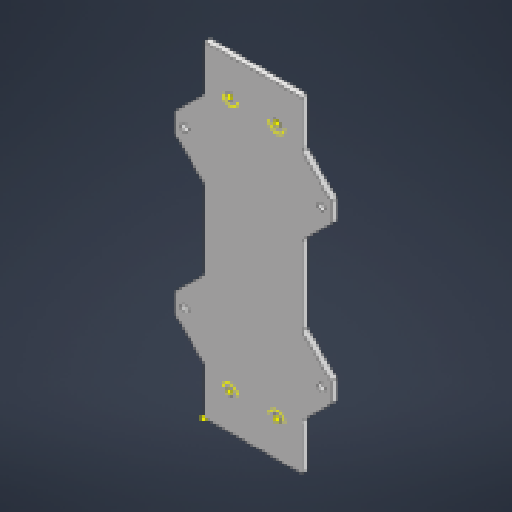
# Autodesk Inventor part: Center_lysekrone
Saved by Autodesk Inventor 2023.4 (Build 274418000, 418)
## iProperties
Created: 2025-10-22
Part Number: Center_lysekrone
Material: Generic
Document SubType Name: Modeling
Designer: Malthe Sennels
Density: 1 g/cm^3
Appearance: Default
Author: Malthe Sennels
Autodesk Inventor part; units mm, degrees
ref_plane "YZ Plane" through (0, 0, 0) normal (1, 0, 0) x (0, 1, 0)
ref_plane "XZ Plane" through (0, 0, 0) normal (0, 1, 0) x (-1, 0, 0)
ref_plane "XY Plane" through (0, 0, 0) normal (0, 0, 1) x (1, 0, 0)
sketch "Sketch1" plane through (0, 0, 0) normal (0, 0, 1) x (1, 0, 0)
  circle A0 centre (37, 149.0522) radius 1.75 projected
  circle A1 centre (13, 149.0522) radius 1.75 projected
  line L0 (50, 167.0522) -> (0, 167.0522) projected
  line L1 (0, 167.0522) -> (0, 157.0522) projected
  line L2 (7.8364, 157.0522) -> (0, 157.0522) construction
  line L3 (9.0389, 148.4955) -> (7.8364, 157.0522) construction
  arc A2 (9.0389, 148.4955) -> (16.9611, 148.4955) centre (13, 149.0522) ccw construction
  line L4 (18.1636, 157.0522) -> (16.9611, 148.4955) construction
  line L5 (31.8364, 157.0522) -> (18.1636, 157.0522) construction
  line L6 (33.0389, 148.4955) -> (31.8364, 157.0522) construction
  arc A3 (33.0389, 148.4955) -> (40.9611, 148.4955) centre (37, 149.0522) ccw construction
  line L7 (42.1636, 157.0522) -> (40.9611, 148.4955) construction
  line L8 (50, 157.0522) -> (42.1636, 157.0522) construction
  line L9 (50, 167.0522) -> (50, 157.0522) projected
  circle A4 centre (13, 18) radius 1.75 projected
  circle A5 centre (37, 18) radius 1.75 projected
  line L10 (0, 0) -> (50, 0) projected
  line L11 (50, 0) -> (50, 10) projected
  line L12 (42.1636, 10) -> (50, 10) construction
  line L13 (40.9611, 18.5567) -> (42.1636, 10) construction
  arc A6 (40.9611, 18.5567) -> (33.0389, 18.5567) centre (37, 18) ccw construction
  line L14 (31.8364, 10) -> (33.0389, 18.5567) construction
  line L15 (18.1636, 10) -> (31.8364, 10) construction
  line L16 (16.9611, 18.5567) -> (18.1636, 10) construction
  arc A7 (16.9611, 18.5567) -> (9.0389, 18.5567) centre (13, 18) ccw construction
  line L17 (7.8364, 10) -> (9.0389, 18.5567) construction
  line L18 (0, 10) -> (7.8364, 10) construction
  line L19 (0, 0) -> (0, 10) projected
  line L20 (0, 167.0522) -> (50, 167.0522)
  line L21 (50, 167.0522) -> (50, 0)
  line L22 (50, 0) -> (0, 0)
  line L23 (0, 0) -> (0, 167.0522)
  constraints: 8 end point, 2 parallel, 1 horizontal, 1 perpendicular
extrude "Extrusion1" add sketch "Sketch1" along normal blind 3
sketch "Sketch2" plane through (0, 0, 3) normal (0, 0, 1) x (1, 0, 0)
  arc A0 (9.0389, 148.4955) -> (16.9611, 148.4955) centre (13, 149.0522) ccw projected
  arc A1 (33.0389, 148.4955) -> (40.9611, 148.4955) centre (37, 149.0522) ccw projected
  arc A2 (40.9611, 18.5567) -> (33.0389, 18.5567) centre (37, 18) ccw projected
  arc A3 (16.9611, 18.5567) -> (9.0389, 18.5567) centre (13, 18) ccw projected
  point P0 (0, 0)
sketch "Sketch3" plane through (0, 0, 0) normal (0, 0, -1) x (-1, 0, 0)
  line L0 (0, 167.0522) -> (0, 0) projected
  line L1 (0, 143.5261) -> (15, 128.5261)
  line L2 (15, 128.5261) -> (15, 118.5261)
  line L3 (15, 118.5261) -> (0, 103.5261)
  line L4 (0, 83.5261) -> (-50, 83.5261) construction
  line L5 (-50, 0) -> (-50, 167.0522) projected
  circle A0 centre (10, 123.5261) radius 1.75
  line L6 (0, 167.0522) -> (0, 0) projected
  line L7 (15, 123.5261) -> (10, 123.5261) construction
  line L8 (-50, 167.0522) -> (0, 167.0522) projected
  line L9 (-25, 167.0522) -> (-25, 0) construction
  line L10 (-50, 143.5261) -> (-65, 128.5261)
  line L11 (-65, 128.5261) -> (-65, 118.5261)
  line L12 (-65, 118.5261) -> (-50, 103.5261)
  circle A1 centre (-60, 123.5261) radius 1.75
  line L13 (0, 23.5261) -> (15, 38.5261)
  line L14 (15, 38.5261) -> (15, 48.5261)
  line L15 (15, 48.5261) -> (0, 63.5261)
  circle A2 centre (10, 43.5261) radius 1.75
  circle A3 centre (-60, 43.5261) radius 1.75
  line L16 (-50, 23.5261) -> (-65, 38.5261)
  line L17 (-65, 38.5261) -> (-65, 48.5261)
  line L18 (-65, 48.5261) -> (-50, 63.5261)
  point P0 (0, 63.5261)
  dimension "d2" = 45
  dimension "d3" = 3.5
  dimension "d4" = 15
  dimension "d5" = 5
  dimension "d6" = 10
  dimension "d7" = 20
  constraints: 30 end point, 15 symmetric about line, 5 midpoint, 4 centre point, 2 point on line, 1 horizontal, 1 parallel, 1 perpendicular, 1 vertical, 3 other
  measures "d2" angle of L0 L3
  measures "d3" diameter of A0
  measures "d4" distance between parallel lines of L2 L0
  measures "d5" distance from line of L2 L7.end
  measures "d6" distance of L1.end L2.end
  measures "d7" distance of L3.end point (0, 83.526)
extrude "Extrusion2" add sketch "Sketch3" against normal up to surface (3 mm away)
ref_plane "Work Plane1" through (25, 63.5261, 0) normal (-1, 0, 0) x (0, 0, 1)
body "Solid1"
